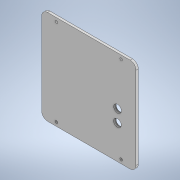
# Autodesk Inventor part: Case_Cover
Saved by Autodesk Inventor 2022 (Build 260153000, 153)
## iProperties
Created: 2024-06-23
Part Number: Case_Cover
Material: Типовые
Document SubType Name: Modeling
Designer: Timur
Density: 1 g/cm^3
Appearance: По умолчанию
Author: Timur
Autodesk Inventor part; units mm, degrees
ref_plane "YZ Plane" through (0, 0, 0) normal (1, 0, 0) x (0, 1, 0)
ref_plane "XZ Plane" through (0, 0, 0) normal (0, 1, 0) x (-1, 0, 0)
ref_plane "XY Plane" through (0, 0, 0) normal (0, 0, 1) x (1, 0, 0)
sketch "Эскиз2" plane through (0, 0, 0) normal (0, 0, 1) x (1, 0, 0)
  line L0 (70, 80) -> (0, 80)
  line L1 (-5, 75) -> (-5, 5)
  line L2 (75, 5) -> (75, 75)
  line L3 (0, 0) -> (70, 0)
  line L4 (70, 73.5411) -> (70, 6.4589)
  line L5 (0, 73.5411) -> (70, 73.5411)
  line L6 (0, 6.4589) -> (0, 73.5411)
  line L7 (70, 6.4589) -> (0, 6.4589)
  arc A0 (8.6686, 75.4679) -> (8.8027, 75.602) centre (7.5, 76.7706) ccw
  circle A1 centre (7.5, 76.7706) radius 1.1
  circle A2 centre (62.5, 76.7706) radius 1.1
  circle A3 centre (62.5, 3.2294) radius 1.1
  circle A4 centre (7.5, 3.2294) radius 1.1
  line L8 (-5, 75) -> (-5, 80)
  line L9 (-5, 80) -> (0, 80)
  line L10 (70, 80) -> (75, 80)
  line L11 (75, 80) -> (75, 75)
  line L12 (75, 5) -> (75, 0)
  line L13 (75, 0) -> (70, 0)
  line L14 (0, 0) -> (-5, 0)
  line L15 (-5, 5) -> (-5, 0)
  circle A5 centre (59.4102, 38.9619) radius 3.25
  circle A6 centre (59.31, 28.4306) radius 3.25
  dimension "d8" = 2.2
  dimension "d9" = 2.2
  dimension "d10" = 2.2
  dimension "d11" = 2.2
  dimension "d12" = 6.5
  dimension "d13" = 6.5
  constraints: 32 end point, 6 centre point, 5 perpendicular, 5 point on line, 2 point on circle, 1 horizontal, 6 other
  measures "d9" diameter of A2
  measures "d10" diameter of A3
  measures "d11" diameter of A4
  measures "d12" diameter of A5
  measures "d13" diameter of A6
extrude "Выдавливание2" add sketch "Эскиз2" along normal blind 2 contours L10 L11 L2 L12 L13 L3 L14 L15 L1 L8 L9 L0 | L4 L7 L6 L5
fillet "Сопряжение2" radius 5 4 edges at (-5, 0, 1) (75, 0, 1) (75, 80, 1) (-5, 80, 1)
